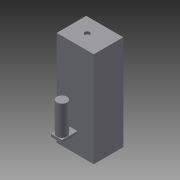
# Autodesk Inventor part: LowerTorso_v2
Saved by Autodesk Inventor 2013 (Build 170138000, 138)
## iProperties
Created: 2012-11-28
Part Number: LowerTorso_v2
Material: Generic
Document SubType Name: Modeling
Designer: Joe
Density: 1 g/cm^3
Author: Joe
Autodesk Inventor part; units mm, degrees
ref_plane "YZ Plane" through (0, 0, 0) normal (1, 0, 0) x (0, 1, 0)
ref_plane "XZ Plane" through (0, 0, 0) normal (0, 1, 0) x (-1, 0, 0)
ref_plane "XY Plane" through (0, 0, 0) normal (0, 0, 1) x (1, 0, 0)
sketch "Sketch1" plane through (0, 0, 0) normal (0, 0, 1) x (1, 0, 0)
  line L0 (0, -69) -> (57, -69)
  line L1 (57, -69) -> (57, 0)
  line L2 (57, 0) -> (117, 0)
  line L3 (117, 0) -> (117, 10)
  line L4 (117, 10) -> (57, 10)
  line L5 (57, 10) -> (57, 298)
  line L6 (57, 298) -> (0, 298)
  line L7 (0, 298) -> (0, -69) construction
  line L8 (0, -69) -> (-57, -69)
  line L9 (-57, -69) -> (-57, 0)
  line L10 (-57, 0) -> (-117, 0)
  line L11 (-117, 0) -> (-117, 10)
  line L12 (-117, 10) -> (-57, 10)
  line L13 (-57, 10) -> (-57, 298)
  line L14 (-57, 298) -> (0, 298)
  point P0 (0, 0)
  dimension "d0" = 57
  dimension "d2" = 10
  dimension "d18" = 367
  dimension "d19" = 117
  dimension "d47" = 69
  constraints: 30 end point, 6 symmetric about line, 5 parallel, 2 collinear, 2 point on line, 1 horizontal, 1 perpendicular
  measures "d0" distance of L5.end L6.end
  measures "d2" distance of L2.end L3.end
  measures "d18" distance between parallel lines of L0 L6
  measures "d19" distance between parallel lines of L3 L7
  measures "d47" distance between parallel lines of L0 L2
extrude "Extrusion1" add sketch "Sketch1" along normal blind 83
sketch "Sketch2" plane through (0, 0, 0) normal (0, 0, -1) x (-1, 0, 0)
  line L0 (57, -69) -> (-57, -69) projected
  line L1 (57, 0) -> (57, -69) projected
  line L2 (117, 0) -> (57, 0) projected
  line L3 (117, 10) -> (117, 0) projected
  line L4 (57, 10) -> (117, 10) projected
  line L5 (57, 298) -> (57, 10) projected
  line L6 (-57, 298) -> (57, 298) projected
  line L7 (-57, 10) -> (-57, 298) projected
  line L8 (-117, 10) -> (-57, 10) projected
  line L9 (-117, 0) -> (-117, 10) projected
  line L10 (-57, 0) -> (-117, 0) projected
  line L11 (-57, -69) -> (-57, 0) projected
  point P0 (0, 0)
extrude "Extrusion2" add sketch "Sketch2" along normal blind 60
sketch "Sketch3" plane through (-57, 298, 83) normal (0, 1, 0) x (1, 0, 0)
  circle A0 centre (57, 82) radius 10
  line L0 (0, 143) -> (114, 143) projected
  line L1 (57, 82) -> (57, 143) construction
  dimension "d10" = 20
  dimension "d51" = 61
  constraints: 2 end point, 1 centre point, 1 midpoint
  measures "d10" diameter of A0
  measures "d51" distance from line of L0 L1.start
extrude "Extrusion3" cut sketch "Sketch3" against normal blind 10
sketch "Sketch4" plane through (-117, 10, 83) normal (0, 1, 0) x (1, 0, 0)
  line L0 (0, 143) -> (60, 143) projected
  line L1 (0, 143) -> (0, 0) projected
  line L2 (21.34, 84) -> (21.34, 143)
  line L3 (118.34, 120.2658) -> (118.34, -20.3509) construction
  line L4 (21.34, 84) -> (118.34, 84) construction
  circle A0 centre (21.34, 84) radius 10
  point P0 (117, 83)
  dimension "d21" = 59
  dimension "d23" = 97
  dimension "d24" = 20
  constraints: 6 end point, 2 parallel, 2 point on line, 1 centre point, 1 coincident, 1 horizontal
  measures "d21" distance of L2.start L2.end
  measures "d23" distance of L2.start L4.end
  measures "d24" diameter of A0
extrude "Extrusion4" cut sketch "Sketch4" against normal through all
mirror "Mirror1" about plane through (0, 0, 0) normal (1, 0, 0) of "Extrusion4"
sketch "Sketch5" plane through (57, 10, 83) normal (0, 1, 0) x (1, 0, 0)
  line L0 (0, 143) -> (0, 0) projected
  line L1 (60, 143) -> (60, 0) projected
  line L2 (60, 143) -> (0, 143)
  line L3 (0, 143) -> (0, 105.1637)
  line L4 (0, 105.1637) -> (60, 105.1637)
  line L5 (60, 105.1637) -> (60, 143)
  line L6 (0, 0) -> (60, 0)
  line L7 (60, 0) -> (60, 62.9414)
  line L8 (60, 62.9414) -> (0, 62.9414)
  line L9 (0, 62.9414) -> (0, 0)
  point P0 (-57, 83)
  constraints: 16 end point, 4 parallel, 2 horizontal, 2 perpendicular, 2 point on line
extrude "Extrusion5" cut sketch "Sketch5" against normal through all contours L2 L1 L4 L0 | L8 L1 L6 L0
mirror "Mirror2" about plane through (0, 0, 0) normal (1, 0, 0) of "Extrusion5"
sketch "Sketch6" plane through (57, 10, -22.1637) normal (0, 1, 0) x (1, 0, 0)
  circle A0 centre (38.66, -21.1637) radius 10 projected
  circle A1 centre (38.66, -21.1637) radius 19.7186
  point P0 (-57, -22.1637)
  constraints: 1 centre point, 1 coincident
extrude "Extrusion6" add sketch "Sketch6" along normal blind 114 contours A0 | A1
mirror "Mirror3" about plane through (0, 0, 0) normal (1, 0, 0) of "Extrusion6"
move or copy body "Move Body3" bodies to move or copy 1 copy no rotation origin (0, 0, 0) rotation axis (0, 1, 0) rotation angle 90
move or copy body "Move Body4" bodies to move or copy 1 copy no rotation origin (0, 0, 0) rotation axis (1, 0, 0) rotation angle 90
move or copy body "Move Body8" bodies to move or copy 1 copy no translate (0, 0, 75)
body "Solid1"
